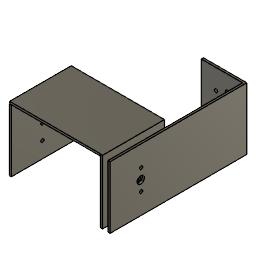
SUPPORT (Autodesk Fusion 360 design; units mm, degrees)
Autodesk Fusion 360 part; units mm, degrees
sketch "Esquisse1" plane through (0, 0, 0) normal (1, 0, 0) x (0, 1, 0)
  line L0 (-100, 50) -> (0, 50)
  line L1 (0, 50) -> (0, -50)
  line L2 (0, -50) -> (-100, -50)
  line L3 (-100, -50) -> (-100, 50)
  constraint horizontal L0
  constraint vertical L1
  constraint horizontal L2
  constraint vertical L3
extrude "Extrusion1" add sketch "Esquisse1" along normal blind 5 makes body 1
sketch "Esquisse2" plane through (5, 0, 0) normal (1, 0, 0) x (0, 1, 0)
sketch "Esquisse3" plane through (0, 0, 0) normal (1, 0, 0) x (0, 1, 0)
  line L0 (-130, 80) -> (0, 80)
  line L1 (0, 80) -> (0, 20)
  line L2 (0, 20) -> (-130, 20)
  line L3 (-130, 20) -> (-130, 80)
  constraint horizontal L0
  constraint vertical L1
  constraint horizontal L2
  constraint vertical L3
extrude "Extrusion2" add sketch "Esquisse3" against normal blind 2 bodies 1
sketch "Esquisse4" plane through (0, 0, 0) normal (1, 0, 0) x (0, 1, 0)
  line L0 (0, 80) -> (2.1401, 80)
  line L1 (2.1401, 80) -> (2.1401, 20)
  line L2 (2.1401, 20) -> (0, 20)
  line L3 (0, 20) -> (0, 80)
  point P0 (0, 80)
  constraint horizontal L0
  constraint vertical L1
  constraint horizontal L2
  constraint vertical L3
  constraint coincident P0 L0.start
extrude "Extrusion3" add sketch "Esquisse4" along normal blind 0 and the other way blind 40 bodies 1
hole "Perçage1" at (-9.7051, 2.1401, 50) direction (0, -1, 0) diameter 13 depth 20 tip angle 118 bodies 1
hole "Perçage2" at (-20, 2.1401, 50) direction (0, -1, 0) diameter 13 depth 20 tip angle 118 bodies 1
hole "Perçage3" at (-14.2643, 2.1401, 50.1489) direction (0, -1, 0) diameter 13 depth 20 tip angle 118 bodies 1
sketch "Esquisse5" plane through (0, 0, 0) normal (0, 1, 0) x (1, 0, 0)
  circle A0 centre (-15, -50) radius 15
  line L0 (-15, -35) -> (-15, -65)
  line L1 (-15, -50) -> (-4.5488, -39.2403)
  line L2 (-15, -50) -> (-4.2403, -60.4512)
  line L3 (-4.2403, -60.4512) -> (-15, -50)
  line L4 (-25.7597, -39.5488) -> (-15, -50)
  line L5 (-15, -50) -> (-25.6661, -60.5468)
  dimension "d18" = 30
  constraint coincident A0 L0.start
  constraint coincident A0 L0.end
  constraint vertical L0
  constraint coincident A0.centre L1.start
  constraint coincident A0 L1.end
  constraint coincident A0 L2.end
  constraint perpendicular L1 L2
  constraint coincident A0 L4.start
  constraint perpendicular L1 L4
  constraint coincident A0 L5.end
  measures "d18" diameter of A0
hole "Perçage4" at (-15, 0, 35) at (-25.7597, 0, 39.5488) at (-4.5488, 0, 39.2403) at (-4.2403, 0, 60.4512) at (-15, 0, 65) at (-25.6661, 0, 60.5468) direction (0, 1, 0) diameter 2 depth 20 tip angle 118 bodies 1
sketch "Esquisse6" plane through (0, 0, 0) normal (0, 1, 0) x (1, 0, 0)
  line L0 (-19.8323, -43.4468) -> (-10, -43.4468)
  line L1 (-10, -43.4468) -> (-13, -49)
  line L2 (-13, -49) -> (-19.8323, -43.4468)
  constraint horizontal L0
extrude "Extrusion4" cut sketch "Esquisse6" along normal blind 5 bodies 1
sketch "Esquisse7" plane through (0, 2.1401, 0) normal (0, 1, 0) x (-1, 0, 0)
  line L0 (0, 80) -> (0, 20)
  line L1 (0, 20) -> (40, 20)
  line L2 (40, 20) -> (40, 80)
  line L3 (40, 80) -> (0, 80)
  line L4 (19.7614, 43.5044) -> (19.8323, 43.4468)
  line L5 (19.8323, 43.4468) -> (10, 43.4468)
  line L6 (10, 43.4468) -> (10.0332, 43.5083)
  arc A0 (11.7861, 56.1579) -> (10.0332, 43.5083) centre (9.7051, 50) ccw
  arc A1 (17.2835, 55.9051) -> (11.7861, 56.1579) centre (14.2643, 50.1489) ccw
  arc A2 (19.7614, 43.5044) -> (17.2835, 55.9051) centre (20, 50) ccw
  circle A3 centre (25.6661, 60.5468) radius 1
  circle A4 centre (4.2403, 60.4512) radius 1
  circle A5 centre (25.7597, 39.5488) radius 1
  circle A6 centre (15, 35) radius 1
  circle A7 centre (4.5488, 39.2403) radius 1
  circle A8 centre (15, 65) radius 1
  line L7 (20.1642, 56.4979) -> (9.7064, 56.5)
  line L8 (20.1642, 56.4979) -> (9.7051, 47.682)
  line L9 (9.7051, 47.682) -> (9.7051, 47.779)
  line L10 (9.7064, 56.5) -> (9.7051, 47.682)
  constraint coincident A2 L7.start
  constraint coincident A0 L7.end
  constraint tangent A0 L7
  constraint perpendicular L7 L9
extrude "Extrusion5" cut sketch "Esquisse7" against normal blind 10 contours A1 A2 L7 bodies 1
sketch "Esquisse8" plane through (0, 2.1401, 0) normal (0, 1, 0) x (-1, 0, 0)
  line L0 (15.6528, 56.4988) -> (19.8383, 56.498)
  arc A0 (19.7614, 43.5044) -> (19.8383, 56.498) centre (20, 50) ccw
  line L1 (19.7614, 43.5044) -> (19.8323, 43.4468)
  line L2 (19.8323, 43.4468) -> (10, 43.4468)
  line L3 (10, 43.4468) -> (10.0332, 43.5083)
  arc A1 (11.7861, 56.1579) -> (10.0332, 43.5083) centre (9.7051, 50) ccw
  arc A2 (15.6528, 56.4988) -> (11.7861, 56.1579) centre (14.2643, 50.1489) ccw
  line L4 (0, 80) -> (0, 20)
  line L5 (0, 20) -> (40, 20)
  line L6 (40, 20) -> (40, 80)
  line L7 (40, 80) -> (0, 80)
  circle A3 centre (25.6661, 60.5468) radius 1
  circle A4 centre (4.2403, 60.4512) radius 1
  circle A5 centre (25.7597, 39.5488) radius 1
  circle A6 centre (15, 35) radius 1
  circle A7 centre (4.5488, 39.2403) radius 1
  circle A8 centre (15, 65) radius 1
  line L8 (19.8383, 56.498) -> (19.7614, 56.498)
  line L9 (19.7614, 56.498) -> (19.7614, 43.5044)
  line L10 (19.7614, 43.5044) -> (19.8383, 43.5044)
  line L11 (19.8383, 43.5044) -> (19.8383, 56.498)
  line L12 (10, 43.4468) -> (19.7614, 43.4468)
  line L13 (19.7614, 43.4468) -> (19.7614, 56.498)
  line L14 (19.7614, 56.498) -> (10, 56.498)
  line L15 (10, 56.498) -> (10, 43.4468)
  constraint horizontal L8
  constraint vertical L9
  constraint horizontal L10
  constraint vertical L11
  constraint coincident A0.start L1.start
  constraint coincident L0.end A0.end
  constraint horizontal L12
  constraint vertical L13
  constraint horizontal L14
  constraint vertical L15
  constraint coincident L2.end L3.start
extrude "Extrusion6" cut sketch "Esquisse8" against normal blind 10 contours A1 A2 L14 L15 bodies 1
delete_face "DeleteFace1" 1 faces at (0, -66.6667, -3.3333) on bodies 1
extrude "Extrusion7" cut 1 faces at (5, -66.6667, 30) along direction (-1, 0, 0) blind 5 on bodies 1 bodies 1
extrude "Extrusion8" add 1 faces at (0, -85.9533, 60) along direction (1, 0, 0) blind 2 on bodies 1 bodies 1
extrude "Extrusion9" cut 1 faces at (-2, -86.6667, 40) along direction (1, 0, 0) blind 2 on bodies 1 bodies 1
sketch "Esquisse9" plane through (0, 2.1401, 0) normal (0, 1, 0) x (-1, 0, 0)
  line L0 (10, 56.498) -> (12.872, 56.498)
  arc A0 (15.6528, 56.4988) -> (12.872, 56.498) centre (14.2643, 50.1489) ccw
  line L1 (15.6528, 56.4988) -> (19.8383, 56.498)
  arc A1 (19.7614, 43.5044) -> (19.8383, 56.498) centre (20, 50) ccw
  line L2 (19.7614, 43.5044) -> (19.8323, 43.4468)
  line L3 (19.8323, 43.4468) -> (10, 43.4468)
  line L4 (10, 43.4468) -> (10.0332, 43.5083)
  arc A2 (10, 56.4933) -> (10.0332, 43.5083) centre (9.7051, 50) ccw
  line L5 (10, 56.4933) -> (10, 56.498)
  line L6 (-2, 20) -> (40, 20)
  line L7 (40, 20) -> (40, 80)
  line L8 (40, 80) -> (-2, 80)
  line L9 (-2, 80) -> (-2, 20)
  circle A3 centre (25.6661, 60.5468) radius 1
  circle A4 centre (4.2403, 60.4512) radius 1
  circle A5 centre (25.7597, 39.5488) radius 1
  circle A6 centre (15, 35) radius 1
  circle A7 centre (4.5488, 39.2403) radius 1
  circle A8 centre (15, 65) radius 1
sketch "Esquisse10" plane through (0, 0, 0) normal (-1, 0, 0) x (0, -1, 0)
  line L0 (0, 20) -> (130, 20)
  line L1 (130, 20) -> (130, 80)
  line L2 (130, 80) -> (0, 80)
  line L3 (0, 80) -> (0, 20)
  line L4 (130, 20) -> (100, 20)
  line L5 (100, 20) -> (100, 80)
  line L6 (100, 80) -> (130, 80)
  line L7 (130, 80) -> (130, 20)
  line L8 (100, 50) -> (130, 50)
  line L9 (130, 50) -> (130, 40)
  line L10 (130, 40) -> (100, 40)
  line L11 (100, 40) -> (100, 50)
  line L12 (130, 60) -> (100, 60)
  line L13 (100, 60) -> (100, 50)
  line L14 (100, 50) -> (130, 50)
  line L15 (130, 50) -> (130, 60)
  constraint horizontal L4
  constraint vertical L5
  constraint horizontal L6
  constraint vertical L7
  constraint coincident L2 L5.end
  constraint coincident L0.end L1.start
  constraint horizontal L8
  constraint vertical L9
  constraint horizontal L10
  constraint vertical L11
  constraint coincident L7 L9.end
  constraint midpoint L5 L8.start
  constraint horizontal L12
  constraint vertical L13
  constraint horizontal L14
  constraint vertical L15
  constraint coincident L7 L12.start
hole "Perçage5" at (0, -99.9937, 40.0782) direction (1, 0, 0) diameter 3 depth 10 tip angle 118 bodies 1
hole "Perçage6" at (0, -100, 60) direction (1, 0, 0) diameter 3 depth 3 tip angle 118 bodies 1
hole "Perçage7" at (-25.7597, 2.1401, 39.5488) direction (0, -1, 0) diameter 3 depth 3 tip angle 118 bodies 1
hole "Perçage8" at (-25.6661, 2.1401, 60.5468) direction (0, -1, 0) diameter 3 depth 3 tip angle 118 bodies 1
hole "Perçage9" at (-4.2403, 2.1401, 60.4512) direction (0, -1, 0) diameter 3 depth 3 tip angle 118 bodies 1
hole "Perçage10" at (-4.5488, 2.1401, 39.2403) direction (0, -1, 0) diameter 3 depth 3 tip angle 118 bodies 1
hole "Perçage11" at (-15, 2.1401, 35) direction (0, -1, 0) diameter 3 depth 3 tip angle 118 bodies 1
hole "Perçage12" at (-15, 2.1401, 65) direction (0, -1, 0) diameter 3 depth 3 tip angle 118 bodies 1
sketch "Esquisse11" plane through (0, 0, 80) normal (0, 0, 1) x (-1, 0, 0)
  line L0 (0, 0) -> (0, 130)
  line L1 (0, 130) -> (-2, 130)
  line L2 (-2, 130) -> (-2, -2.1401)
  line L3 (-2, -2.1401) -> (40, -2.1401)
  line L4 (40, -2.1401) -> (40, 0)
  line L5 (40, 0) -> (0, 0)
  line L6 (0, 100) -> (100.1298, 100)
  line L7 (100.1298, 100) -> (100.1298, 0)
  line L8 (100.1298, 0) -> (0, 0)
  line L9 (0, 0) -> (0, 100)
  line L10 (10, 130) -> (100.1298, 130)
  line L11 (100.1298, 130) -> (100.1298, 70.3583)
  line L12 (100.1298, 70.3583) -> (10, 70.3583)
  line L13 (10, 70.3583) -> (10, 130)
  constraint horizontal L6
  constraint vertical L7
  constraint horizontal L8
  constraint vertical L9
  constraint coincident L0 L6.start
  constraint horizontal L10
  constraint vertical L11
  constraint horizontal L12
  constraint vertical L13
  constraint coincident L7 L11.end
extrude "Extrusion10" add sketch "Esquisse11" along normal blind 2 separate body contours L6 L10 L11 L13 | L6 L7 L11 L12 L13 makes body 2
sketch "Esquisse12" plane through (0, -70.3583, 0) normal (0, 1, 0) x (-1, 0, 0)
  line L0 (10, 80) -> (100.1298, 80)
  line L1 (100.1298, 80) -> (100.1298, 82)
  line L2 (100.1298, 82) -> (10, 82)
  line L3 (10, 82) -> (10, 80)
  line L4 (100, 20) -> (98, 20)
  line L5 (98, 20) -> (98, 80)
  line L6 (98, 80) -> (100, 80)
  line L7 (100, 80) -> (100, 20)
  dimension "d60" = 2
  constraint horizontal L4
  constraint vertical L5
  constraint horizontal L6
  constraint vertical L7
  measures "d60" distance of L4.start L4.end
extrude "Extrusion11" add sketch "Esquisse12" against normal blind 60 contours L0 L4 L5 L6 L7 bodies 2
sketch "Esquisse13" plane through (-10, 0, 0) normal (1, 0, 0) x (0, 1, 0)
  line L0 (-130, 80) -> (-70.3583, 80)
  line L1 (-70.3583, 80) -> (-70.3583, 82)
  line L2 (-70.3583, 82) -> (-130, 82)
  line L3 (-130, 82) -> (-130, 80)
  line L4 (-70.3583, 82) -> (-130.3678, 82)
  line L5 (-130.3678, 82) -> (-130.3678, 20.3349)
  line L6 (-130.3678, 20.3349) -> (-70.3583, 20.3349)
  line L7 (-70.3583, 20.3349) -> (-70.3583, 82)
  constraint horizontal L4
  constraint vertical L5
  constraint horizontal L6
  constraint vertical L7
  constraint coincident L1.end L2.start
extrude "Extrusion12" add sketch "Esquisse13" against normal blind 2 contours L0 L3 L4 L5 L6 L7 bodies 2
sketch "Esquisse14" plane through (0, -130.3678, 0) normal (0, -1, 0) x (1, 0, 0)
hole "Perçage13" at (-10, -100.3631, 35.8369) direction (-1, 0, 0) diameter 13 depth 3 tip angle 118 bodies 2
hole "Perçage14" at (-10, -100.3631, 51.1675) direction (-1, 0, 0) diameter 13 depth 3 tip angle 118 bodies 2
hole "Perçage15" at (-10, -100.3631, 43.3656) direction (-1, 0, 0) diameter 13 depth 3 tip angle 118 bodies 2
sketch "Esquisse15" plane through (-10, 0, 0) normal (1, 0, 0) x (0, 1, 0)
  arc A0 (-105.5624, 47.2665) -> (-105.6621, 39.6013) centre (-100.3631, 43.3656) ccw
  arc A1 (-95.1638, 47.2665) -> (-105.5624, 47.2665) centre (-100.3631, 51.1675) ccw
  arc A2 (-95.064, 39.6013) -> (-95.1638, 47.2665) centre (-100.3631, 43.3656) ccw
  arc A3 (-105.6621, 39.6013) -> (-95.064, 39.6013) centre (-100.3631, 35.8369) ccw
  line L0 (-70.3583, 20.3349) -> (-70.3583, 82)
  line L1 (-70.3583, 82) -> (-130.3678, 82)
  line L2 (-130.3678, 82) -> (-130.3678, 20.3349)
  line L3 (-130.3678, 20.3349) -> (-70.3583, 20.3349)
  line L4 (-106.8624, 51.2634) -> (-93.9763, 51.2634)
  line L5 (-93.9763, 51.2634) -> (-93.9763, 34.6291)
  line L6 (-93.9763, 34.6291) -> (-106.8624, 34.6291)
  line L7 (-106.8624, 34.6291) -> (-106.8624, 51.2634)
  constraint horizontal L4
  constraint vertical L5
  constraint horizontal L6
  constraint vertical L7
  constraint coincident A3 L5.end
  constraint coincident A1 L4.start
extrude "Extrusion13" cut sketch "Esquisse15" against normal blind 5 contours A0 A1 L7 | A0 A3 L7 | A1 A2 L5 | A2 A3 L5 bodies 2
sketch "Esquisse16" plane through (0, -130.3678, 0) normal (0, -1, 0) x (1, 0, 0)
hole "Perçage16" at (-100, -100.3583, 50) direction (1, 0, 0) diameter 3 depth 3 tip angle 118 bodies 2
hole "Perçage17" at (-98, -100.3631, 35.3582) direction (-1, 0, 0) diameter 3 depth 3 tip angle 118 bodies 2
hole "Perçage18" at (-100, -100.3109, 64.238) direction (1, 0, 0) diameter 3 depth 20 tip angle 118 bodies 2
sketch "Esquisse17" plane through (0, 0, 0) normal (1, 0, 0) x (0, 1, 0)
hole "Perçage19" at (-10, -110.8035, 53.2714) direction (-1, 0, 0) diameter 3 depth 5 tip angle 118 bodies 2
hole "Perçage20" at (-10, -89.902, 53.2259) direction (-1, 0, 0) diameter 3 depth 5 tip angle 118 bodies 2
hole "Perçage21" at (-10, -85.3683, 42.6551) direction (-1, 0, 0) diameter 3 depth 5 tip angle 118 bodies 2
hole "Perçage22" at (-10, -89.902, 31.7541) direction (-1, 0, 0) diameter 3 depth 5 tip angle 118 bodies 2
hole "Perçage23" at (-10, -110.914, 31.8189) direction (-1, 0, 0) diameter 3 depth 5 tip angle 118 bodies 2
hole "Perçage24" at (-10, -115.3651, 42.6492) direction (-1, 0, 0) diameter 3 depth 5 tip angle 118 bodies 2
hole "Perçage25" at (2, -100.3725, 49.9842) direction (-1, 0, 0) diameter 7 depth 3 tip angle 118 bodies 1
move_body "Déplacer1" bodies 2 to x (1, 0, 0) y (0, 1, 0) z (0, 0, 1) at (5, 0, 0)
